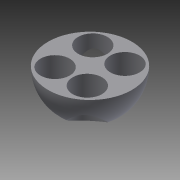
# Autodesk Inventor part: SentiBot botton
Saved by Autodesk Inventor 2015 (Build 190159000, 159)
## iProperties
Created: 2015-07-02
Part Number: SentiBot botton
Material: Generic
Document SubType Name: Modeling
Designer: Sudhar
Density: 1 g/cm^3
Appearance: Default
Author: Sudhar
Autodesk Inventor part; units mm, degrees
ref_plane "YZ Plane" through (0, 0, 0) normal (1, 0, 0) x (0, 1, 0)
ref_plane "XZ Plane" through (0, 0, 0) normal (0, 1, 0) x (-1, 0, 0)
ref_plane "XY Plane" through (0, 0, 0) normal (0, 0, 1) x (1, 0, 0)
sketch "Sketch1" plane through (0, 0, 0) normal (0, 0, 1) x (1, 0, 0)
  arc A0 (-2.9756, -24.1911) -> (22.4244, 1.2089) centre (-2.9756, 1.2089) ccw
  line L0 (-2.9756, 1.2089) -> (-2.9756, -24.1911)
  line L1 (-2.9756, 1.2089) -> (22.4244, 1.2089)
  dimension "d0" = 50.8
  constraints: 4 end point, 2 point on circle, 1 centre point, 1 perpendicular, 1 vertical
  measures "d0" diameter of A0
revolve "Revolution1" add sketch "Sketch1" angle 360 about axis through (-2.9756, 1.2089, 0) along (0, -1, 0)
sketch "Sketch2" plane through (-2.9756, 1.2089, 0) normal (0, 1, 0) x (1, 0, 0)
  line L0 (12.0985, 11.6032) -> (-0.4296, 11.6032)
  line L1 (12.0985, 11.6032) -> (12.0985, 2.9428)
  circle A0 centre (-9.9233, 11.6032) radius 8.89
  circle A1 centre (9.6347, 11.6032) radius 8.89
  circle A2 centre (-9.9233, -11.2568) radius 8.89
  circle A3 centre (9.6347, -11.2568) radius 8.89
  dimension "d4" = 20.1422
  dimension "d7" = 23.2918
  dimension "d22" = 17.78
  dimension "d25" = 19.558
  dimension "d28" = 22.86
  constraints: 4 centre point, 4 end point, 3 horizontal, 3 vertical, 6 other
  measures "d22" diameter of A0
  measures "d25" distance of A0.centre A1.centre
  measures "d28" distance of A0.centre A2.centre
extrude "Extrusion1" cut sketch "Sketch2" against normal blind 25.4
sketch "Sketch3" plane through (0, 0, 0) normal (0, 0, 1) x (1, 0, 0)
  line L0 (-2.7068, 20.711) -> (-2.7068, -36.5415)
  constraints: 2 end point, 1 vertical
shell "Shell1" thickness 1.016 removed faces 0
body "Solid1"
